Autodesk Inventor part; units mm, degrees
(part 2 of 2)
sketch "Sketch10" plane through (0, 0, 9.3) normal (0, 0, 1) x (1, 0, 0)
  arc A0 (3, -24.6) -> (1.5, -23.1) centre (1.5, -24.6) ccw construction
  line L0 (0, -23.1) -> (1.5, -23.1) construction
  line L1 (0, -33.2811) -> (0, -23.1) construction
  spline S0 degree 2 poles (0, -33.2811) (1.2955, -35.1685) (0, -37.056) knots 0 0 0 1 1 1 weights 1 1.375 1 construction
  line L2 (0, -41.3315) -> (0, -37.056) construction
  line L3 (3, -24.6) -> (3, -29.7467) construction
  line L4 (8.9062, -65.3371) -> (8.9062, -65.8371)
  line L5 (13.0938, -65.8371) -> (8.9062, -65.8371)
  line L6 (13.0938, -65.8371) -> (13.0938, -65.3371)
  line L7 (13.0938, -65.3371) -> (15.9062, -65.3371)
  line L8 (15.9062, -65.3371) -> (15.9062, -65.8371)
  line L9 (23.1, -65.8371) -> (15.9062, -65.8371)
  line L10 (23.1, -6.5) -> (23.1, -65.8371)
  line L11 (27.4, -6.5) -> (23.1, -6.5)
  line L12 (27.4, 0) -> (27.4, -6.5)
  line L13 (0, 0) -> (27.4, 0)
  line L14 (0, -1) -> (0, 0)
  line L15 (2.5, -1) -> (0, -1)
  line L16 (2.5, -17.5) -> (2.5, -1)
  line L17 (0, -17.5) -> (2.5, -17.5)
  line L18 (0, -65.8371) -> (0, -17.5)
  line L19 (6.0938, -65.8371) -> (0, -65.8371)
  line L20 (6.0938, -65.8371) -> (6.0938, -65.3371)
  line L21 (6.0938, -65.3371) -> (8.9062, -65.3371)
  arc A1 (4.0542, -29.6883) -> (19.4959, -28.2768) centre (12.35, -35.2722) ccw
  arc A2 (9.7, -14.6801) -> (4.0542, -29.6883) centre (9.2226, -23.0665) ccw
  arc A3 (16.7181, -19.2746) -> (9.7, -14.6801) centre (14.7, -14.7) ccw
  arc A4 (17.618, -23.3446) -> (16.7181, -19.2746) centre (9.2226, -23.0665) ccw
  circle A5 centre (1.5356, -30.0714) radius 1
  circle A6 centre (1.5, -41.3315) radius 1
  circle A7 centre (1.5356, -30.0714) radius 2
  circle A8 centre (1.5, -41.3315) radius 2
  circle A9 centre (4, -46.5095) radius 3.5
  arc A10 (4.0542, -29.6883) -> (16.9384, -26.387) centre (12.35, -35.2722) ccw
  arc A11 (9.7, -14.6801) -> (4.0542, -29.6883) centre (9.2226, -23.0665) ccw
  circle A12 centre (1.5, -41.3315) radius 2.25
  arc A13 (3, -41.3315) -> (0, -41.3315) centre (1.5, -41.3315) ccw
  line L22 (3, -30.3961) -> (3, -41.3315)
  arc A14 (3, -29.7467) -> (3, -30.3961) centre (1.5356, -30.0714) ccw
  arc A15 (19.3256, -22.3566) -> (17.618, -23.3446) centre (19.8907, -25.3029) ccw
  arc A16 (20.9964, -22.5141) -> (19.3256, -22.3566) centre (20.3569, -20.3569) ccw
  arc A17 (19.4959, -28.2768) -> (20.9964, -22.5141) centre (19.8907, -25.3029) ccw
  point P0 (0, 0)
  dimension "d145" = 2
  dimension "d146" = 2
  dimension "d147" = 4
  dimension "d148" = 4
  dimension "d149" = 7
  dimension "d150" = 1.5
  dimension "d151" = 1.5
  dimension "d152" = 4.5
  constraints: 6 centre point, 3 coincident, 3 tangent
  measures "d145" diameter of A5
  measures "d146" diameter of A6
  measures "d147" diameter of A7
  measures "d148" diameter of A8
  measures "d149" diameter of A9
  measures "d150" distance from line of L3 A6.centre
  measures "d151" distance from line of L2 A6.centre
  measures "d152" diameter of A12
hole "Hole7" at (1.5356, -30.0714, 9.3) at (1.5, -41.3315, 9.3) direction (0, 0, -1) diameter 2 end through all clearance for "Countersunk Flat Head Screw ISO 2009/7046" size "M2" standard "ISO"
sketch "Sketch11" plane through (2.5, -17.5, 0) normal (-1, 0, 0) x (0, 0, 1)
  circle A0 centre (6, 7) radius 1.25 projected
  point P0 (0, 17.5)
hole "Hole8" at (2.5, -10.5, 6) direction (1, 0, 0) diameter 3 depth 4 counterbore diameter 3.5 counterbore depth 0.5
body "Solid2"
